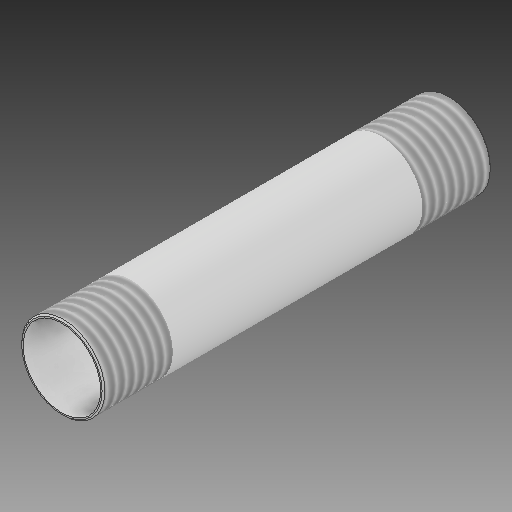
# Autodesk Inventor part: VerteilerLuft1
Saved by Autodesk Inventor 2021 (Build 250183000, 183)
## iProperties
Created: 2021-10-22
Part Number: VerteilerLuft1
Material: Generisch
Document SubType Name: Modeling
Designer: lukas
Density: 1 g/cm^3
Appearance: Vorgabe
Stock Number: Verteiler 1
Author: lukas
Autodesk Inventor part; units mm, degrees
ref_plane "XZ Plane" through (0, 0, 0) normal (0, 1, 0) x (-1, 0, 0)
ref_plane "XY Plane" through (0, 0, 0) normal (0, 0, 1) x (1, 0, 0)
sketch "Skizze1" plane through (0, 0, 0) normal (0, 0, 1) x (1, 0, 0)
  line L0 (-21, 0) -> (21, 0) projected
  line L1 (0, -21) -> (0, 21) projected
  circle A0 centre (0, 0) radius 15
  circle A1 centre (0, 0) radius 14
  dimension "d0" = 30
  dimension "d1" = 28
  constraints: 2 centre point, 2 coincident
  measures "d0" diameter of A0
  measures "d1" diameter of A1
extrude "Extrusion1" add sketch "Skizze1" against normal blind 140 contours A1 L1 A0 L0 | L0 A0 L1 A1 | A1 L0 A0 L1 | L1 A0 L0 A1
thread "Gewinde1" size "M30x3.5" class "6g" standard "ANSI Metric M Profile" length 25
thread "Gewinde2" size "M30x3.5" class "6g" standard "ANSI Metric M Profile" length 25
chamfer "Fase1" distance 0.5 angle 45 1 edges at (-15, 0, 0)
chamfer "Fase2" distance 0.5 angle 45 1 edges at (-15, 0, -140)
ref_plane "Arbeitsebene1" through (15, 0, 0) normal (1, 0, 0) x (0, 1, 0)
sketch "Skizze2" plane through (0, 0, 0) normal (1, 0, 0) x (0, 1, 0)
  line L0 (15, -0.5) -> (-15, -0.5) projected
  line L1 (14.5, -140) -> (-14.5, -140) projected
  line L2 (-14.5, 0) -> (14.5, 0) projected
  point P0 (0, 0)
  point P1 (0, -40)
  point P2 (0, -55)
  point P3 (0, -70)
  point P4 (0, -85)
  point P5 (0, -100)
  dimension "d17" = 40
  dimension "d18" = 15
  dimension "d19" = 15
  dimension "d20" = 15
  dimension "d21" = 40
  dimension "d22" = 15
  measures "d17" distance from line of L1 point (0, -100)
  measures "d18" distance of point (0, -55) point (0, -40)
  measures "d19" distance of point (0, -70) point (0, -55)
  measures "d20" distance of point (0, -85) point (0, -100)
  measures "d21" distance from line of point (0, -40) L2
  measures "d22" distance of point (0, -85) point (0, -70)
hole "Bohrung1" at (0, 0, -40) at (0, 0, -55) at (0, 0, -70) at (0, 0, -85) at (0, 0, -100) direction (-1, 0, 0) diameter 11.445 end through all thread size "G13.157x1.337" designation "G 1/4" standard "ISO Pipe Threads"
